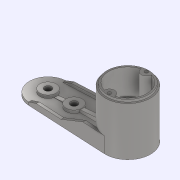
# Autodesk Inventor part: pt1
Saved by Autodesk Inventor 2021 (Build 250183000, 183)
## iProperties
Created: 2021-10-15
Part Number: pt1
Material: Stainless Steel
Document SubType Name: Modeling
Designer: DuctopwH
Density: 8 g/cm^3
Appearance: Semi-Polished
Author: DuctopwH
Autodesk Inventor part; units mm, degrees
ref_plane "YZ Plane" through (0, 0, 0) normal (1, 0, 0) x (0, 1, 0)
ref_plane "XZ Plane" through (0, 0, 0) normal (0, 1, 0) x (-1, 0, 0)
sketch "Sketch1" plane through (0, 0, 0) normal (0, 1, 0) x (-1, 0, 0)
  circle A0 centre (0, 0) radius 19.5
  line L0 (0, 0) -> (69, 0) construction
  circle A1 centre (69, 0) radius 16
  line L1 (69.8116, -15.9794) -> (0.9891, -19.4749)
  line L2 (69.8116, 15.9794) -> (0.9891, 19.4749)
  point P0 (0.9891, 19.4749)
  dimension "d0" = 39
  dimension "d1" = 32
  dimension "d2" = 69
  constraints: 6 end point, 2 coincident, 2 symmetric about line, 1 horizontal, 8 other
  measures "d2" distance of point (0, 0) L0.end
extrude "Extrusion1" add sketch "Sketch1" along normal blind 2.5 contours A0 L2 A1 L1 | A1
sketch "Sketch3" plane through (0, 0, 0) normal (0, 0, 1) x (1, 0, 0)
  line L0 (0, 0) -> (0, 29.1077)
  line L1 (0, 22) -> (-16.5, 22)
  line L2 (-16.5, 22) -> (-16.5, 44)
  line L3 (-16.5, 44) -> (-19.5, 44)
  line L4 (-19.5, 44) -> (-19.5, 2.5)
  line L5 (-19.5, 2.5) -> (-0.9891, 2.5) projected
  line L6 (-19.5, 2.5) -> (-19.5, 0)
  line L7 (-19.5, 0) -> (-16.5, 0)
  line L8 (-19.5, 0) -> (-0.9891, 0) projected
  line L9 (-16.5, 0) -> (-16.5, 18)
  line L10 (-16.5, 18) -> (0, 18)
  line L11 (-18, 44) -> (-18, 42)
  line L12 (-18, 42) -> (-19.5, 42)
  line L13 (-4, 18) -> (-4, 19)
  line L14 (-4, 19) -> (-11, 19)
  line L15 (-11, 19) -> (-11, 22)
  point P0 (-16.5, 2.5)
  dimension "d5" = 44
  dimension "d6" = 2
  dimension "d7" = 18
  dimension "d8" = 16.5
  dimension "d10" = 4
  dimension "d11" = 3
  dimension "d12" = 22
  dimension "d13" = 11
  dimension "d14" = 1
  constraints: 28 end point, 7 perpendicular, 6 point on line, 5 vertical, 1 collinear, 1 horizontal, 1 midpoint
  measures "d5" distance between parallel lines of L3 L7
  measures "d6" distance between parallel lines of L3 L12
  measures "d7" distance between parallel lines of L0 L11
  measures "d8" distance between parallel lines of L0 L2
  measures "d10" distance between parallel lines of L0 L13
  measures "d11" distance between parallel lines of L1 L14
  measures "d12" distance between parallel lines of L3 L1
  measures "d13" distance between parallel lines of L0 L15
  measures "d14" distance between parallel lines of L14 L10
revolve "Revolution1" add sketch "Sketch3" angle 360 about axis through (0, 0, 0) along (0, 1, 0) contours L10 L9 L5 L4 L12 L11 L3 L2 L1 L15 L14 L13 | L9 L7 L6 L5
sketch "Sketch4" plane through (0, 2.5, 0) normal (0, 1, 0) x (1, 0, 0)
  line L0 (0, 0) -> (-85, 0)
  arc A0 (-69.8116, 15.9794) -> (-69.8116, -15.9794) centre (-69, 0) ccw projected
  circle A1 centre (-46.5, 0) radius 7
  circle A2 centre (-69, 0) radius 7
  dimension "d17" = 46.5
  dimension "d18" = 22.5
  dimension "d19" = 14
  constraints: 2 centre point, 2 end point, 2 point on line, 1 equal radius, 1 horizontal, 1 point on circle
  measures "d17" distance of L0.start A1.centre
  measures "d18" distance of A2.centre A1.centre
  measures "d19" diameter of A2
extrude "Extrusion2" add sketch "Sketch4" along normal blind 2.5
ref_plane "Work Plane1" through (-69.6848, 0, 13.4826) normal (-0.0507, 0, 0.9987) x (0.9987, 0, 0.0507)
sketch "Sketch6" plane through (-69.6848, 0, 13.4826) normal (-0.0507, 0, 0.9987) x (0.9987, 0, 0.0507)
  line L0 (68.9112, 0) -> (68.9112, 13.5)
  line L1 (68.9112, 13.5) -> (49.4112, 13.5)
  line L2 (49.4112, 13.5) -> (29.471, 5)
  line L3 (29.471, 5) -> (7, 5)
  line L4 (7, 5) -> (0, 2.5)
  line L5 (66.9355, 2.5) -> (-1.6211, 2.5) projected
  line L6 (29.471, 2.5) -> (29.471, 5) projected
  line L7 (7, 2.5) -> (7, 5) projected
  line L8 (49.4112, 2.5) -> (49.4112, 42) projected
  line L9 (7, 5) -> (-7, 5) projected
  line L10 (0, 5) -> (0, 18.3194) construction
  line L11 (66.9355, 0) -> (-1.6211, 0) projected
  line L12 (66.9355, 2.5) -> (68.9112, 2.5)
  dimension "d23" = 13.5
  dimension "d24" = 5
  constraints: 14 end point, 6 point on line, 2 perpendicular, 2 vertical, 1 horizontal, 1 midpoint
  measures "d23" distance of L0.start L0.end
  measures "d24" distance between parallel lines of L11 L3
extrude "Extrusion3" add sketch "Sketch6" along normal blind 2.5
mirror "Mirror1" about plane through (0, 0, 0) normal (0, 0, 1) of "Extrusion3"
sketch "Sketch7" plane through (0, 0, 0) normal (0, 0, 1) x (1, 0, 0)
  line L0 (-17.1617, 6.6953) -> (-62, 2.52)
  line L1 (-62, 2.5) -> (-62, 5) projected
  line L2 (-62, 2.52) -> (-62, 2.5)
  line L3 (-10.4025, 2.5) -> (-69.6848, 2.5) projected
  line L4 (-17.1617, 2.5) -> (-62, 2.5)
  line L5 (-17.1617, 2.5) -> (-17.1617, 6.6953)
  line L6 (-0.9891, 0) -> (-69.8116, 0) projected
  line L7 (-62, 2.52) -> (-62.2148, 2.5)
  point P0 (0, 0)
  dimension "d27" = 5.32
  dimension "d28" = 2.52
  constraints: 10 end point, 3 point on line, 2 vertical, 1 collinear, 1 perpendicular
  measures "d27" angle of L0 L3
  measures "d28" distance from line of L6 L0.end
extrude "Extrusion4" add sketch "Sketch7" along normal mid plane 3.5
sketch "Sketch8" plane through (-46.5, 5, 0) normal (0, 1, 0) x (1, 0, 0)
  arc A0 (-6.7777, -1.75) -> (6.7777, -1.75) centre (0, 0) ccw projected
  circle A1 centre (0, 0) radius 3
  arc A2 (-15.7148, 1.7207) -> (-15.7148, -1.7207) centre (-22.5, 0) ccw projected
  circle A3 centre (-22.5, 0) radius 3
  point P0 (46.5, 0)
  point P1 (-15.5, 0)
  dimension "d31" = 6
  constraints: 2 centre point, 2 coincident, 1 equal radius
  measures "d31" diameter of A1
extrude "Extrusion5" cut sketch "Sketch8" against normal through all
sketch "Sketch9" plane through (0, 44, 0) normal (0, 1, 0) x (1, 0, 0)
  circle A0 centre (0, -16) radius 4.5
  line L0 (0, 0) -> (24.199, 0) construction
  circle A1 centre (0, 0) radius 16.5 projected
  circle A2 centre (0, 16) radius 4.5
  point P0 (-4.4983, 15.875)
  point P1 (4.4983, 15.875)
  point P2 (-4.4983, -15.875)
  point P3 (4.4983, -15.875)
  dimension "d34" = 9
  dimension "d35" = 16
  constraints: 2 centre point, 2 end point, 1 horizontal, 1 symmetric about line, 1 vertical alignment, 1 other
  measures "d34" diameter of A0
  measures "d35" distance from line of L0 A0.centre
extrude "Extrusion6" add sketch "Sketch9" against normal up to surface (22 mm away) contours A1 A0 | A1 A2 picked at (-0.1776, -14.7973) picked at (-0.1776, 14.7973)
sketch "Sketch10" plane through (0, 44, 0) normal (0, 1, 0) x (1, 0, 0)
  arc A0 (4.4983, -15.875) -> (-4.4983, -15.875) centre (0, -16) ccw projected
  circle A1 centre (0, -16) radius 1.5
  line L0 (0, 0) -> (9.3395, 0) construction
  circle A2 centre (0, 16) radius 1.5
  dimension "d38" = 3
  constraints: 2 centre point, 2 end point, 1 coincident, 1 horizontal, 1 symmetric about line, 1 other
  measures "d38" diameter of A1
extrude "Extrusion7" cut sketch "Sketch10" against normal blind 4
sketch "Sketch11" plane through (0, 0, 0) normal (0, -1, 0) x (1, 0, 0)
  circle A0 centre (0, 16) radius 1.5 projected
  circle A1 centre (0, 16) radius 2.5
  line L0 (0, 0) -> (10.318, 0)
  circle A2 centre (0, -16) radius 2.5
  dimension "d41" = 5
  constraints: 2 centre point, 2 end point, 1 coincident, 1 horizontal, 1 symmetric about line, 1 other
  measures "d41" diameter of A1
extrude "Extrusion8" cut sketch "Sketch11" against normal up to surface (40 mm away) contours A0 | A1 | A2
sketch "Sketch12" plane through (0, 44, 0) normal (0, 1, 0) x (1, 0, 0)
  line L0 (36.079, 0) -> (-96.4154, 0)
  line L1 (-96.4154, 0) -> (-96.4154, 28.1723)
  line L2 (-96.4154, 28.1723) -> (36.079, 28.1723)
  line L3 (36.079, 28.1723) -> (36.079, 0)
  point P0 (0, 0)
  constraints: 8 end point, 2 parallel, 1 horizontal, 1 perpendicular
body "Solid1"
